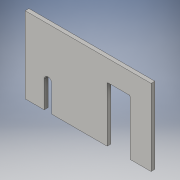
# Autodesk Inventor part: InsideWall
Saved by Autodesk Inventor 2016 (Build 200138000, 138)
## iProperties
Created: 2016-05-26
Part Number: InsideWall
Material: Generic
Document SubType Name: Modeling
Designer: cutrones
Density: 1 g/cm^3
Appearance: Default
Author: cutrones
Autodesk Inventor part; units mm, degrees
ref_plane "YZ Plane" through (0, 0, 0) normal (1, 0, 0) x (0, 1, 0)
ref_plane "XZ Plane" through (0, 0, 0) normal (0, 1, 0) x (-1, 0, 0)
ref_plane "XY Plane" through (0, 0, 0) normal (0, 0, 1) x (1, 0, 0)
sketch "Sketch1" plane through (0, 0, 0) normal (0, 0, 1) x (1, 0, 0)
  line L0 (0, 0) -> (419.1, 0)
  line L1 (419.1, 0) -> (419.1, 254)
  line L2 (419.1, 254) -> (0, 254)
  line L3 (0, 254) -> (0, 0)
  line L4 (273.05, 184.15) -> (349.25, 184.15)
  line L5 (349.25, 184.15) -> (349.25, 0)
  line L6 (349.25, 0) -> (273.05, 0)
  line L7 (273.05, 0) -> (273.05, 184.15)
  circle A0 centre (76.2, 88.9) radius 12.7
  line L8 (63.5, 88.9) -> (88.9, 88.9)
  line L9 (88.9, 88.9) -> (88.9, 0)
  line L10 (88.9, 0) -> (63.5, 0)
  line L11 (63.5, 0) -> (63.5, 88.9)
  dimension "d5" = 25.4
  dimension "d0" = 419.1
  dimension "d1" = 254
  dimension "d2" = 76.2
  dimension "d3" = 184.15
  dimension "d4" = 273.05
  dimension "d6" = 88.9
  dimension "d7" = 63.5
  dimension "d8" = 25.4
  dimension "d9" = 76.2
  constraints: 24 end point, 6 parallel, 3 horizontal, 3 perpendicular, 2 point on line, 1 horizontal alignment, 2 other
  measures "d0" distance of L1.end L2.end
  measures "d1" distance of L0.end L1.end
  measures "d2" distance of L4.start L4.end
  measures "d3" distance of L6.end L4.start
  measures "d4" distance between parallel lines of L7 L3
  measures "d6" distance of L10.end L8.start
  measures "d7" distance between parallel lines of L11 L3
  measures "d8" distance between parallel lines of L9 L11
  measures "d9" distance from line of L3 point (76.2, 88.9)
extrude "Extrusion1" add sketch "Sketch1" along normal mid plane 12.7 contours L3 L2 L1 L0 L5 L4 L7 L9 A0 L11
fillet "Fillet1" radius 3.175 1 edges at (273.05, 184.15, 0)
fillet "Fillet2" radius 3.175 1 edges at (349.25, 184.15, 0)
equation "\"d0\" = Length"
equation "\"d1\" = Height"
equation "\"d10\" = Thick"
equation "\"Length\" = 419.1"
equation "\"Height\" = 254"
equation "\"Thick\" = 12.7"
body "Solid1"
